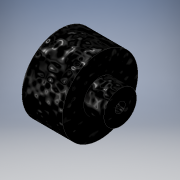
# Autodesk Inventor part: 60mm Mecanum Wheel
Saved by Autodesk Inventor 2019.4 (Build 234330000, 330)
## iProperties
Created: 2020-01-31
Part Number: 60mm Mecanum Wheel
Material: Generic
Document SubType Name: Modeling
Designer: admin
Mass: 87.5 g
Surface Area: 140.995 cm^2
Volume: 96.56 cm^3
Density: 0.906172 g/cm^3
Appearance: Black
Author: admin
Autodesk Inventor part; units mm, degrees
ref_plane "YZ Plane" through (0, 0, 0) normal (1, 0, 0) x (0, 1, 0)
ref_plane "XZ Plane" through (0, 0, 0) normal (0, 1, 0) x (-1, 0, 0)
ref_plane "XY Plane" through (0, 0, 0) normal (0, 0, 1) x (1, 0, 0)
sketch "Sketch1" plane through (0, 0, 0) normal (0, 0, 1) x (1, 0, 0)
  line L0 (0, 0) -> (0, 30)
  line L1 (0, 30) -> (32, 30)
  line L2 (32, 30) -> (32, 13)
  line L3 (32, 13) -> (48, 13)
  line L4 (48, 13) -> (48, 4)
  line L5 (48, 4) -> (0, 4)
  line L6 (0, 0) -> (80.4021, 0)
  dimension "d0" = 30
  dimension "d1" = 32
  dimension "d2" = 16
  dimension "d3" = 4
  dimension "d4" = 13
  constraints: 14 end point, 4 perpendicular, 2 vertical, 1 horizontal, 1 point on line
  measures "d0" distance of L0.start L0.end
  measures "d1" distance of L0.end L1.end
  measures "d2" distance of L2.end L3.end
  measures "d3" distance from line of L0.start L5
  measures "d4" distance from line of L0.start L3
revolve "Revolution1" add sketch "Sketch1" angle 360 about axis through (0, 0, 0) along (1, 0, 0)
body "Solid1"
